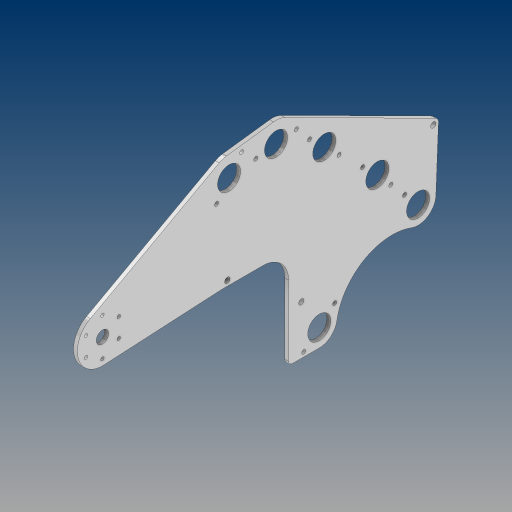
# Autodesk Inventor part: Intake Roller Plate
Saved by Autodesk Inventor 2024.3 (Build 283343000, 343)
## iProperties
Created: 2024-07-25
Part Number: Intake Roller Plate
Material: Aluminum 6061
Document SubType Name: Modeling
Designer: Kenji
Density: 2.7 g/cm^3
Appearance: Aluminum - Dark
Author: Kenji
Autodesk Inventor part; units mm, degrees
ref_plane "YZ Plane" through (0, 0, 0) normal (1, 0, 0) x (0, 1, 0)
ref_plane "XZ Plane" through (0, 0, 0) normal (0, 1, 0) x (-1, 0, 0)
ref_plane "XY Plane" through (0, 0, 0) normal (0, 0, 1) x (1, 0, 0)
sketch "Sketch1" plane through (0, 0, 0) normal (1, 0, 0) x (0, 1, 0)
  line L0 (127, 0) -> (127, -31.75) construction
  line L1 (95.25, -63.5) -> (31.75, -63.5) construction
  line L2 (0, -31.75) -> (0, 0) construction
  arc A0 (95.25, -63.5) -> (127, -31.75) centre (95.25, -31.75) ccw construction
  arc A1 (0, -31.75) -> (31.75, -63.5) centre (31.75, -31.75) ccw construction
  line L3 (0, 0) -> (0, 19.05) construction
  line L4 (0, 19.05) -> (-12.7, 19.05) construction
  line L5 (82.55, 19.05) -> (82.55, 292.1) construction
  circle A2 centre (82.55, 292.1) radius 25.4 construction
  circle A3 centre (82.55, 292.1) radius 31.75 construction
  circle A4 centre (231.775, 292.1) radius 25.4 construction
  circle A5 centre (231.775, 292.1) radius 31.75 construction
  line L6 (-12.7, 19.05) -> (82.55, 19.05) construction
  line L7 (127, 0) -> (0, 0) construction
  line L8 (-12.7, 19.05) -> (-12.7, -285.75) construction
  circle A6 centre (38.1, -175.1237) radius 50.8 construction
  circle A7 centre (96.0971, -224.5481) radius 25.4 construction
  circle A8 centre (96.0971, -224.5481) radius 14.2875
  circle A9 centre (153.6466, -173.8737) radius 25.4 construction
  circle A10 centre (153.6466, -173.8737) radius 14.2875
  circle A11 centre (249.9155, -47.8338) radius 22.225 construction
  circle A12 centre (249.9155, -47.8338) radius 25.4 construction
  circle A13 centre (249.9155, -47.8338) radius 14.2875
  line L9 (82.55, 19.05) -> (127, 19.05) construction
  line L10 (127, 19.05) -> (127, 0) construction
  circle A14 centre (153.6466, -173.8737) radius 22.225 construction
  circle A15 centre (96.0971, -224.5481) radius 22.225 construction
  circle A16 centre (25.4, -101.6) radius 25.4 construction
  circle A17 centre (25.4, -101.6) radius 23.8125 construction
  line L11 (25.4, -76.2) -> (25.4, -63.5) construction
  circle A18 centre (216.5234, -107.8815) radius 25.4 construction
  circle A19 centre (216.5234, -107.8815) radius 22.225 construction
  circle A20 centre (216.5234, -107.8815) radius 14.2875
  line L12 (0, -101.6) -> (-12.7, -101.6) construction
  circle A21 centre (64.1171, -79.375) radius 6.477 construction
  circle A22 centre (25.4, -101.6) radius 14.2875
  circle A23 centre (64.1171, -79.375) radius 3.2512
  circle A24 centre (84.9265, -149.1714) radius 50.8 construction
  circle A25 centre (144.1337, -98.2698) radius 50.8 construction
  circle A26 centre (105.5334, -118.9394) radius 50.8 construction
  circle A27 centre (172.6204, -243.5219) radius 3.2512
  circle A28 centre (242.5281, 10.5862) radius 14.2875
  circle A29 centre (242.5281, 10.5862) radius 22.225 construction
  line L13 (216.5234, -107.8815) -> (153.6466, -173.8737) construction
  line L14 (153.6466, -173.8737) -> (96.0971, -224.5481) construction
  line L15 (82.55, 19.05) -> (31.75, 19.05) construction
  line L16 (31.75, 19.05) -> (31.75, 292.1) construction
  line L17 (31.75, 292.1) -> (82.55, 292.1) construction
  circle A30 centre (242.5281, 10.5862) radius 7.62 construction
  line L18 (-12.7, -285.75) -> (571.5, -285.75) construction
  line L19 (571.5, -285.75) -> (571.5, 292.1) construction
  line L20 (31.75, 292.1) -> (571.5, 292.1) construction
  line L21 (127, 19.05) -> (571.5, 19.05) construction
  circle A31 centre (149.9325, 168.1327) radius 7.62
  circle A32 centre (149.9325, 168.1327) radius 23.495 construction
  circle A33 centre (173.4275, 168.1327) radius 2.0828
  circle A34 centre (149.9325, 168.1327) radius 27.94 construction
  circle A35 centre (149.9325, 168.1327) radius 31.115 construction
  circle A36 centre (161.68, 188.4799) radius 2.0828
  circle A37 centre (138.185, 188.4799) radius 2.0828
  circle A38 centre (126.4375, 168.1327) radius 2.0828
  circle A39 centre (138.185, 147.7854) radius 2.0828
  circle A40 centre (161.68, 147.7854) radius 2.0828
  line L22 (-12.7, -63.5) -> (368.3, -63.5) construction
  circle A41 centre (172.6204, -243.5219) radius 6.4262 construction
  line L23 (368.3, -63.5) -> (368.3, -285.75) construction
  line L24 (7.043, -116.7676) -> (81.9407, -207.4149) construction
  circle A42 centre (64.1171, -79.375) radius 6.35 construction
  circle A43 centre (242.5281, 10.5862) radius 25.4 construction
  line L25 (242.5281, 10.5862) -> (249.9155, -47.8338) construction
  line L26 (82.55, 19.05) -> (141.3002, 19.05) construction
  line L27 (141.3002, 19.05) -> (141.3002, 209.55) construction
  line L28 (141.3002, 209.55) -> (82.55, 209.55) construction
  line L29 (82.55, 209.55) -> (82.55, 19.05) construction
  circle A44 centre (133.35, 12.7) radius 6.35 construction
  circle A45 centre (177.072, -42.6893) radius 50.8 construction
  circle A46 centre (177.8, -23.221) radius 50.8 construction
  circle A47 centre (25.4, -101.6) radius 22.225 construction
  line L30 (267.7274, 13.7727) -> (275.1148, -44.6473)
  line L31 (178.36, -246.4121) -> (272.6017, -59.2575)
  line L32 (3.175, -101.6) -> (3.175, -68.2752)
  circle A48 centre (133.35, 12.7) radius 3.2512
  line L33 (177.2374, 183.052) -> (264.8178, 22.7652)
  arc A49 (267.7274, 13.7727) -> (264.8178, 22.7652) centre (242.5281, 10.5862) ccw
  arc A50 (272.6017, -59.2575) -> (275.1148, -44.6473) centre (249.9155, -47.8338) ccw
  arc A51 (172.6204, -249.9481) -> (178.36, -246.4121) centre (172.6204, -243.5219) ccw
  arc A52 (3.175, -101.6) -> (21.6232, -123.5017) centre (25.4, -101.6) ccw
  arc A53 (7.9502, -63.5) -> (3.175, -68.2752) centre (7.9502, -68.2752) ccw
  arc A54 (177.2374, 183.052) -> (118.8648, 166.4176) centre (149.9325, 168.1327) ccw
  line L34 (127, -31.75) -> (127, 19.05)
  line L35 (127, 19.05) -> (118.8648, 166.4176)
  line L36 (141.3002, 53.086) -> (157.9626, 53.086) construction
  line L37 (157.9626, 53.086) -> (157.9626, 86.106) construction
  line L38 (157.9626, 86.106) -> (141.3002, 86.106) construction
  line L39 (141.3002, 86.106) -> (141.3002, 53.086) construction
  line L40 (249.9155, -47.8338) -> (253.1021, -73.0332) construction
  line L41 (249.9155, -47.8338) -> (246.729, -22.6345) construction
  circle A55 centre (246.729, -22.6345) radius 2.4257
  circle A56 centre (253.1021, -73.0332) radius 2.4257
  line L42 (242.5281, 10.5862) -> (262.5999, -4.9792) construction
  line L43 (242.5281, 10.5862) -> (222.4562, 26.1515) construction
  circle A57 centre (262.5999, -4.9792) radius 2.4257
  circle A58 centre (222.4562, 26.1515) radius 2.4257
  circle A59 centre (262.5999, -4.9792) radius 5.6007 construction
  circle A60 centre (222.4562, 26.1515) radius 5.6007 construction
  circle A61 centre (246.729, -22.6345) radius 5.6007 construction
  circle A62 centre (253.1021, -73.0332) radius 5.6007 construction
  line L44 (216.5234, -107.8815) -> (234.0446, -89.4922) construction
  line L45 (216.5234, -107.8815) -> (199.0022, -126.2709) construction
  circle A63 centre (234.0446, -89.4922) radius 2.4257
  circle A64 centre (199.0022, -126.2709) radius 2.4257
  circle A65 centre (171.1678, -155.4844) radius 2.4257
  circle A66 centre (134.5835, -190.6594) radius 2.4257
  arc A67 (75.2683, -216.795) -> (95.1813, -246.7543) centre (96.0971, -224.5481) ccw
  circle A68 centre (8.7757, -82.396) radius 2.4257
  circle A69 centre (8.7757, -82.396) radius 5.6007 construction
  arc A70 (75.2683, -216.795) -> (21.6232, -123.5017) centre (9.7416, -192.4039) ccw
  line L46 (8.7757, -82.396) -> (42.0243, -120.804) construction
  circle A71 centre (42.0243, -120.804) radius 2.4257
  circle A72 centre (42.0243, -120.804) radius 5.6007 construction
  line L47 (7.9502, -63.5) -> (95.25, -63.5)
  arc A73 (95.25, -63.5) -> (127, -31.75) centre (95.25, -31.75) ccw
  line L48 (172.6204, -249.9481) -> (95.1813, -246.7543)
  circle A74 centre (115.1602, -207.7624) radius 2.4257
  line L49 (96.0971, -224.5481) -> (77.0341, -241.3339) construction
  line L50 (135.0132, 195.4376) -> (295.3, 283.0179) construction
  line L51 (299.0152, 145.2002) -> (151.6476, 137.065) construction
  arc A75 (381.5652, 113.4502) -> (349.8152, 145.2002) centre (349.8152, 113.4502) ccw construction
  line L52 (419.6652, 21.3752) -> (386.3404, 21.3752) construction
  arc A76 (381.5652, 26.1504) -> (386.3404, 21.3752) centre (386.3404, 26.1504) ccw construction
  line L53 (381.5652, 26.1504) -> (381.5652, 113.4502) construction
  line L54 (349.8152, 145.2002) -> (299.0152, 145.2002) construction
  circle A77 centre (305.3652, 151.5502) radius 6.35 construction
  circle A78 centre (307.479, 260.7282) radius 25.4 construction
  circle A79 centre (365.899, 268.1157) radius 25.4 construction
  circle A80 centre (425.9467, 234.7235) radius 25.4 construction
  circle A81 centre (491.9389, 171.8467) radius 25.4 construction
  circle A82 centre (561.5871, 190.8205) radius 6.4262 construction
  circle A83 centre (542.6133, 114.2973) radius 25.4 construction
  line L55 (568.0133, 190.8205) -> (564.8194, 113.3814) construction
  arc A84 (534.8602, 93.4685) -> (564.8194, 113.3814) centre (542.6133, 114.2973) ccw construction
  arc A85 (534.8602, 93.4685) -> (441.5669, 39.8234) centre (510.469, 27.9418) ccw construction
  line L56 (564.4773, 196.5601) -> (377.3226, 290.8018) construction
  arc A86 (568.0133, 190.8205) -> (564.4773, 196.5601) centre (561.5871, 190.8205) ccw construction
  line L57 (304.2925, 285.9276) -> (362.7125, 293.315) construction
  arc A87 (377.3226, 290.8018) -> (362.7125, 293.315) centre (365.899, 268.1157) ccw construction
  arc A88 (304.2925, 285.9276) -> (295.3, 283.0179) centre (307.479, 260.7282) ccw construction
  arc A89 (419.6652, 21.3752) -> (441.5669, 39.8234) centre (419.6652, 43.6002) ccw construction
  circle A90 centre (419.6652, 43.6002) radius 25.4 construction
  line L58 (82.55, 133.35) -> (88.9, 133.35) construction
  line L59 (82.55, 184.15) -> (88.9, 184.15) construction
  point P0 (-12.7, -175.1237)
  point P1 (179.0466, -173.8737)
  point P2 (104.775, 19.05)
  point P3 (179.0466, -243.5219)
  point P4 (127, -63.5)
  point P5 (3.175, -63.5)
  point P6 (96.0971, -249.9481)
  point P7 (381.5652, 21.3752)
  point P8 (323.0444, 280.8001)
  point P9 (291.9136, 240.6564)
  point P10 (391.0983, 271.3022)
  point P11 (340.6997, 264.9291)
  point P12 (407.5574, 252.2447)
  point P13 (444.3361, 217.2023)
  point P14 (491.9389, 197.2467)
  point P15 (473.5496, 189.3679)
  point P16 (508.7246, 152.7837)
  point P17 (561.5871, 197.2467)
  point P18 (568.0133, 114.2973)
  point P19 (525.8276, 133.3603)
  point P20 (559.399, 95.2342)
  point P21 (394.2652, 43.6002)
  point P22 (419.6652, 18.2002)
  point P23 (400.4612, 26.9759)
  point P24 (438.8692, 60.2245)
  dimension "d58" = 101.6
  dimension "d284" = 46.99
  dimension "d2" = 31.75
  dimension "d3" = 19.05
  dimension "d4" = 12.7
  dimension "d7" = 273.05
  dimension "d8" = 50.8
  dimension "d9" = 6.35
  dimension "d10" = 50.8
  dimension "d11" = 6.35
  dimension "d12" = 149.225
  dimension "d14" = 127
  dimension "d16" = 304.8
  dimension "d175" = 31.75
  dimension "d180" = 50.8
  dimension "d181" = 1.5875
  dimension "d187" = 31.75
  dimension "d189" = 12.7
  dimension "d191" = 12.954
  dimension "d192" = 28.575
  dimension "d201" = 6.5024
  dimension "d207" = 101.6
  dimension "d208" = 101.6
  dimension "d210" = 130.175
  dimension "d214" = 15.875
  dimension "d218" = 6.5024
  dimension "d220" = 143.1895
  dimension "d236" = 50.8
  dimension "d237" = 44.45
  dimension "d267" = 15.24
  dimension "d271" = 584.2
  dimension "d283" = 15.24
  dimension "d285" = 4.1656
  dimension "d290" = 55.88
  dimension "d292" = 3.175
  dimension "d321" = 360
  dimension "d323" = 381
  dimension "d328" = 3.175
  dimension "d336" = 12.7
  dimension "d375" = 12.7
  dimension "d376" = 108.7971
  dimension "d377" = 76.6801
  dimension "d388" = 50.8
  dimension "d389" = 3.175
  dimension "d395" = 44.45
  dimension "d399" = 58.7502
  dimension "d400" = 190.5
  dimension "d404" = 12.7
  dimension "d405" = 101.6
  dimension "d406" = 101.6
  dimension "d407" = 58.42
  dimension "d409" = 3.175
  dimension "d410" = 6.5024
  dimension "d411" = 4.7752
  dimension "d427" = 16.6624
  dimension "d428" = 33.02
  dimension "d429" = 34.036
  dimension "d433" = 4.8514
  dimension "d434" = 4.8514
  dimension "d435" = 4.8514
  dimension "d436" = 4.8514
  dimension "d437" = 3.175
  dimension "d438" = 3.175
  dimension "d439" = 3.175
  dimension "d440" = 3.175
  dimension "d441" = 45
  constraints: 121 end point, 91 point on circle, 88 centre point, 35 tangent, 23 point on line, 21 coincident, 19 equal radius, 15 perpendicular, 8 concentric, 8 horizontal alignment, 8 parallel, 6 collinear, 6 horizontal, 4 vertical, 3 vertical alignment, 2 midpoint, 99 other
  measures "d2" radius of A0
  measures "d3" distance of L2.end L3.end
  measures "d4" distance of L3.end L4.end
  measures "d7" distance of L5.start L5.end
  measures "d8" diameter of A2
  measures "d9" radial gap between concentric circles of A2 A3
  measures "d10" diameter of A4
  measures "d11" radial gap between concentric circles of A4 A5
  measures "d12" distance of L17.end A4.centre
  measures "d14" distance of L0.start L2.end
  measures "d16" distance of L4.end L8.end
  measures "d175" radius of A1
  measures "d180" diameter of A16
  measures "d187" distance of L0.start L0.end
  measures "d189" distance of L12.start L12.end
  measures "d191" diameter of A21
  measures "d192" diameter of A22
  measures "d201" diameter of A23
  measures "d207" diameter of A24
  measures "d208" diameter of A25
  measures "d210" distance of A21.centre A14.centre
  measures "d214" distance from line of L1 A21.centre
  measures "d218" diameter of A27
  measures "d220" distance of A0.centre A19.centre
  measures "d236" distance of L5.start L15.end
  measures "d237" distance of L4.end L15.end
  measures "d267" diameter of A30
  measures "d271" distance of L8.end L18.end
  measures "d283" diameter of A31
  measures "d285" diameter of A33
  measures "d290" diameter of A34
  measures "d292" radial gap between concentric circles of A34 A35
  measures "d323" distance of L22.start L22.end
  measures "d328" radial gap between concentric circles of A27 A41
  measures "d336" diameter of A42
  measures "d375" distance of L11.start L11.end
  measures "d376" distance from line of L8 A15.centre
  measures "d377" distance of L13.end L14.end
  measures "d388" diameter of A9
  measures "d389" radial gap between concentric circles of A15 A7
  measures "d395" diameter of A15
  measures "d399" distance of L28.end L27.end
  measures "d400" distance of L27.end L26.end
  measures "d404" diameter of A44
  measures "d405" diameter of A45
  measures "d406" diameter of A46
  measures "d407" vertical distance of L25.start L25.end
  measures "d409" radial gap between concentric circles of A16 A47
  measures "d410" diameter of A48
  measures "d411" radius of A53
  measures "d427" distance of L38.end L37.end
  measures "d428" distance between parallel lines of L36 L38
  measures "d429" distance from line of L26.end L36
  measures "d433" diameter of A55
  measures "d434" diameter of A56
  measures "d435" diameter of A57
  measures "d436" diameter of A58
  measures "d437" radial gap between concentric circles of A57 A59
  measures "d438" radial gap between concentric circles of A58 A60
  measures "d439" radial gap between concentric circles of A55 A61
  measures "d440" radial gap between concentric circles of A56 A62
  measures "d441" angle of L25 L42
extrude "Extrusion10" add sketch "Sketch1" along normal blind 4.7625
body "Solid9"
